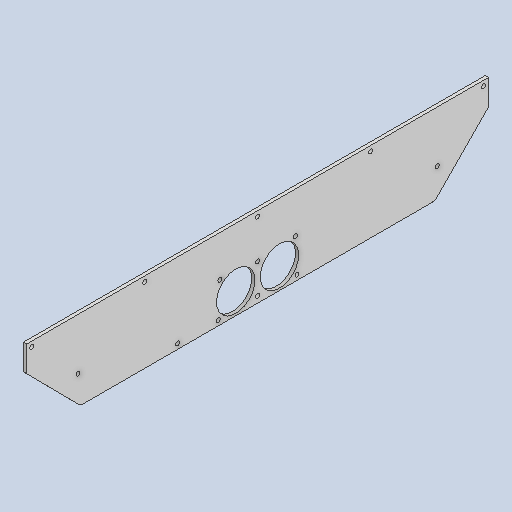
# Autodesk Inventor part: insideChassiPlate2.0
Saved by Autodesk Inventor 2023 (Build 270158000, 158)
## iProperties
Created: 2022-09-08
Part Number: insideChassiPlate2.0
Material: Generic
Document SubType Name: Modeling
Designer: deli
Density: 1 g/cm^3
Appearance: Default
Author: deli
Autodesk Inventor part; units mm, degrees
ref_plane "YZ Plane" through (0, 0, 0) normal (1, 0, 0) x (0, 1, 0)
ref_plane "XZ Plane" through (0, 0, 0) normal (0, 1, 0) x (-1, 0, 0)
ref_plane "XY Plane" through (0, 0, 0) normal (0, 0, 1) x (1, 0, 0)
sketch "Sketch1" plane through (0, 0, 0) normal (1, 0, 0) x (0, 1, 0)
  arc A0 (-110.5167, 35.6829) -> (-112.0027, 32.1259) centre (-107.0027, 32.1259) ccw projected
  line L0 (-112.0027, 32.1259) -> (-112.0027, -308.9783) projected
  arc A1 (-112.0027, -308.9783) -> (-110.5167, -312.5353) centre (-107.0027, -308.9783) ccw projected
  line L1 (-110.5167, -312.5353) -> (-59.0027, -363.4262) projected
  line L2 (-59.0027, -363.4262) -> (-34.0027, -363.4262) projected
  line L3 (-34.0027, -363.4262) -> (-34.0027, 86.5738) projected
  line L4 (-34.0027, 86.5738) -> (-59.0027, 86.5738) projected
  line L5 (-59.0027, 86.5738) -> (-110.5167, 35.6829) projected
  circle A2 centre (-107.0027, -60.5173) radius 2 projected
  circle A3 centre (-39.0027, -138.4262) radius 2 projected
  circle A4 centre (-73.8579, -101.7083) radius 2 projected
  circle A5 centre (-39.0027, 81.5738) radius 2 projected
  circle A6 centre (-73.8579, -175.1441) radius 2 projected
  circle A7 centre (-107.0027, -176.8201) radius 2 projected
  circle A8 centre (-107.0027, -100.0323) radius 2 projected
  circle A9 centre (-105.7353, -138.4262) radius 2 projected
  circle A10 centre (-76.7702, -138.4262) radius 2 projected
  circle A11 centre (-91.2527, -159.7175) radius 7 construction
  circle A12 centre (-91.2527, -117.135) radius 7 construction
  circle A13 centre (-39.0027, -358.4262) radius 2 projected
  circle A14 centre (-39.0027, -28.4262) radius 2 projected
  circle A15 centre (-39.0027, -248.4262) radius 2 projected
  circle A16 centre (-84.0027, -313.4262) radius 2 projected
  circle A17 centre (-84.0027, 36.5738) radius 2 projected
  circle A18 centre (-91.2527, -117.135) radius 18.75
  circle A19 centre (-91.2527, -159.7175) radius 18.75
  point P0 (0, 0)
  dimension "d0" = 37.5
  dimension "d1" = 37.5
  constraints: 2 centre point, 2 coincident
  measures "d0" diameter of A18
  measures "d1" diameter of A19
extrude "Extrusion1" add sketch "Sketch1" along normal blind 3.175
equation "\"d1\" = d0"
body "Solid1"
